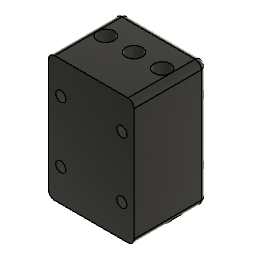
Front Idler Bottom v11 (Autodesk Fusion 360 archive; units mm, degrees)
design "Z Bearing Block"
Autodesk Fusion 360 part; units mm, degrees
sketch "Sketch1" plane through (0, 0, 0) normal (0, 1, 0) x (1, 0, 0)
  line L0 (-14, -20.5) -> (14, -20.5)
  line L1 (14, -20.5) -> (14, 20.5)
  line L2 (14, 20.5) -> (-14, 20.5)
  line L3 (-14, 20.5) -> (-14, -20.5)
  line L4 (-14, -20.5) -> (14, 20.5) construction
  line L5 (14, -20.5) -> (-14, 20.5) construction
  line L6 (-10, 10) -> (10, 10) construction
  line L7 (10, 10) -> (10, -10) construction
  line L8 (10, -10) -> (-10, -10) construction
  line L9 (-10, -10) -> (-10, 10) construction
  line L10 (-10, 10) -> (10, -10) construction
  line L11 (10, 10) -> (-10, -10) construction
  circle A0 centre (10, -10) radius 1.65
  circle A1 centre (10, 10) radius 1.65
  circle A2 centre (-10, -10) radius 1.65
  circle A3 centre (-10, 10) radius 1.65
  circle A4 centre (10, -10) radius 3
  circle A5 centre (-10, -10) radius 3
  circle A6 centre (10, 10) radius 3
  circle A7 centre (-10, 10) radius 3
  dimension "d1" = 28
  dimension "d2" = 41
  dimension "d3" = 20
  dimension "d4" = 20
  dimension "d5" = 3.3
  dimension "d6" = 3.3
  dimension "d7" = 3.3
  dimension "d8" = 3.3
  dimension "d9" = 6
  dimension "d10" = 6
  dimension "d11" = 6
  dimension "d12" = 6
  constraint horizontal L0
  constraint perpendicular L0 L1
  constraint parallel L0 L2
  constraint parallel L1 L3
  constraint coincident L4 origin
  constraint coincident L5 origin
  constraint horizontal L6
  constraint perpendicular L6 L7
  constraint parallel L6 L8
  constraint parallel L7 L9
  constraint coincident L10 origin
  constraint coincident L11 origin
  constraint coincident L7.end L8.start
  constraint coincident L6.end L7.start
  constraint coincident L8.end L9.start
  constraint coincident L6.start L9.end
  constraint concentric A0 A4
  constraint concentric A2 A5
  constraint concentric A1 A6
  constraint concentric A3 A7
  measures "d1" distance of L1.end L2.end
  measures "d2" distance of L0.end L1.end
  measures "d3" distance of L7.end L8.end
  measures "d4" distance of L6.end L7.end
  measures "d5" diameter of A0
  measures "d6" diameter of A1
  measures "d7" diameter of A2
  measures "d8" diameter of A3
  measures "d9" diameter of A4
  measures "d10" diameter of A5
  measures "d11" diameter of A6
  measures "d12" diameter of A7
extrude "Extrude1" add sketch "Sketch1" along normal blind 24 contours L0 L1 L2 L3 | A4 | A5 | A6 | A7
extrude "Extrude2" cut sketch "Sketch1" against normal blind 3 from surface at 24 contours A4 | A5 | A6 | A7
sketch "Sketch2" plane through (0, 0, 20.5) normal (0, 0, 1) x (-1, 0, 0)
  line L0 (14, 0) -> (-14, 0)
  line L1 (-14, 0) -> (-14, -24)
  line L2 (-14, -24) -> (14, -24)
  line L3 (14, -24) -> (14, 0)
  line L4 (-14, 0) -> (-14, -24)
  line L5 (14, 0) -> (-14, 0)
  line L6 (14, -24) -> (-14, -24)
  line L7 (14, 0) -> (14, -24)
  line L8 (-11.65, -21) -> (-8.35, -21)
  line L9 (-8.35, 0) -> (-11.65, 0)
  line L10 (8.35, -21) -> (11.65, -21)
  line L11 (11.65, 0) -> (8.35, 0)
  line L12 (-11.65, 0) -> (-8.35, 0) construction
  line L13 (-8.35, 0) -> (-8.35, -21) construction
  line L14 (-8.35, -21) -> (-11.65, -21) construction
  line L15 (-11.65, -21) -> (-11.65, 0) construction
  line L16 (8.35, -21) -> (11.65, -21) construction
  line L17 (11.65, -21) -> (11.65, 0) construction
  line L18 (11.65, 0) -> (8.35, 0) construction
  line L19 (8.35, 0) -> (8.35, -21) construction
  line L20 (14, 0) -> (-14, 0) construction
  line L21 (-14, 0) -> (-14, -13.98) construction
  line L22 (-14, -13.98) -> (14, -13.98) construction
  line L23 (14, -13.98) -> (14, 0) construction
  line L24 (14, 0) -> (-14, -13.98) construction
  line L25 (-14, 0) -> (14, -13.98) construction
  circle A0 centre (-9.25, -13.98) radius 4.5
  circle A1 centre (0, -13.98) radius 4.5
  circle A2 centre (9.25, -13.98) radius 4.5
  circle A3 centre (-9.25, -13.98) radius 2.7
  circle A4 centre (0, -13.98) radius 2.7
  circle A5 centre (9.25, -13.98) radius 2.7
  line L26 (-14, -13.98) -> (-13.75, -13.98) construction
  line L27 (-4.75, -13.98) -> (-4.5, -13.98) construction
  line L28 (4.5, -13.98) -> (4.75, -13.98) construction
  line L29 (13.75, -13.98) -> (14, -13.98) construction
  point P0 (0, -6.99)
  dimension "d28" = 13.98
  dimension "d29" = 9
  dimension "d30" = 9
  dimension "d31" = 9
  dimension "d32" = 5.4
  dimension "d33" = 5.4
  dimension "d34" = 5.4
  constraint horizontal L12
  constraint vertical L13
  constraint horizontal L14
  constraint vertical L15
  constraint coincident L8.end L13.end
  constraint coincident L9.end L12.start
  constraint horizontal L16
  constraint vertical L17
  constraint horizontal L18
  constraint vertical L19
  constraint coincident L11.start L17.end
  constraint coincident L10.start L16.start
  constraint horizontal L20
  constraint perpendicular L20 L21
  constraint parallel L20 L22
  constraint parallel L21 L23
  constraint coincident L24 P0
  constraint coincident L25 P0
  constraint coincident L0.end L1.start
  constraint coincident L0.start L3.end
  constraint horizontal L26
  constraint coincident L22 A0.centre
  constraint coincident L22 A1.centre
  constraint coincident L22 A2.centre
  constraint horizontal L27
  constraint horizontal L28
  constraint collinear L27 L28
  constraint collinear L26 L27
  constraint coincident L22 L21.end
  constraint equal L26 L27
  constraint equal L27 L28
  constraint coincident A2 L28.end
  constraint coincident A1 L28.start
  constraint coincident A1 L27.end
  constraint coincident A0 L27.start
  constraint coincident A0 L26.end
  constraint horizontal L29
  constraint collinear L28 L29
  constraint equal L28 L29
  constraint coincident A2 L29.start
  constraint coincident L23 L22.end
  constraint coincident L21 L22.start
  constraint coincident A0.centre A3.centre
  constraint coincident A1.centre A4.centre
  constraint coincident A2.centre A5.centre
  measures "d28" distance of L0.end L21.end
  measures "d29" diameter of A0
  measures "d30" diameter of A1
  measures "d31" diameter of A2
  measures "d32" diameter of A3
  measures "d33" diameter of A4
  measures "d34" diameter of A5
extrude "Extrude5" cut sketch "Sketch2" against normal blind 41 contours A4
extrude "Extrude6" cut sketch "Sketch2" against normal blind 5 contours A3 | A5
extrude "Extrude7" cut sketch "Sketch2" against normal blind 36 from surface at -5 contours A0 | A2 | A3 | A5
fillet "Fillet1" radius 2 8 edges at (0, 24, 20.5) (14, 12, 20.5) (14, 12, -20.5) (0, 24, -20.5) (14, 24, 0) (-14, 24, 0) (-14, 12, 20.5) (-14, 12, -20.5)
extrude "Extrude8" cut sketch "Sketch2" along normal blind 5 from surface at -41 contours A1
